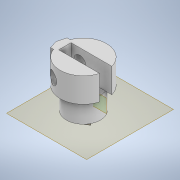
# Autodesk Inventor part: handle_base
Saved by Autodesk Inventor 2021 (Build 250183000, 183)
## iProperties
Created: 2021-03-06
Part Number: handle_base
Material: Generic
Document SubType Name: Modeling
Designer: ben
Density: 1 g/cm^3
Appearance: Default
Mass: 193.865 g
Surface Area: 332.78 cm^2
Volume: 193.865 cm^3
Author: ben
Autodesk Inventor part; units mm, degrees
ref_plane "YZ Plane" through (0, 0, 0) normal (1, 0, 0) x (0, 1, 0)
ref_plane "XZ Plane" through (0, 0, 0) normal (0, 1, 0) x (-1, 0, 0)
ref_plane "XY Plane" through (0, 0, 0) normal (0, 0, 1) x (1, 0, 0)
ref_plane "Work Plane1" through (-35, 22.5, -35) normal (0, 0, 1) x (1, 0, 0)
sketch "Sketch1" plane through (-35, 22.5, -35) normal (0, 0, 1) x (1, 0, 0)
  circle A0 centre (35, -42) radius 27.5
  circle A1 centre (35, -42) radius 6
  point P0 (35, -22.5)
  dimension "d0" = 55
  dimension "d24" = 12
  constraints: 2 centre point, 1 coincident
  measures "d0" diameter of A0
  measures "d24" diameter of A1
ref_plane "Work Plane2" through (0, -19.5, 0) normal (0, 0, 1) x (1, 0, 0)
sketch "Sketch2" plane through (0, -19.5, 0) normal (0, 0, 1) x (1, 0, 0)
  arc A0 (-36.1421, -10) -> (-36.1421, 10) centre (0, 0) ccw
  line L0 (30, -10) -> (-36.1421, -10)
  line L1 (-36.1421, 10) -> (30, 10)
  line L2 (30, 10) -> (30, -10)
  line L3 (34.9857, -13.5) -> (39.9857, -13.5)
  line L4 (39.9857, -13.5) -> (39.9857, 13.5)
  line L5 (39.9857, 13.5) -> (34.9857, 13.5)
  line L6 (34.9857, 13.5) -> (34.9857, -13.5)
  line L7 (39.9857, -13.5) -> (43.6938, 0)
  line L8 (43.6938, 0) -> (39.9857, 13.5)
  point P0 (0, 19.5)
  dimension "d3" = 75
  dimension "d40" = 5
  dimension "d41" = 27
  dimension "d44" = 14
  constraints: 18 end point, 4 horizontal, 4 point on circle, 3 parallel, 1 centre point, 1 perpendicular, 1 vertical, 1 other
  measures "d3" diameter of A0
  measures "d40" distance of L3.start L3.end
  measures "d41" distance of L5.end L3.start
  measures "d44" distance of L3.end L7.end
extrude "Extrusion2" add sketch "Sketch2" along normal blind 40
ref_plane "Work Plane3" through (-36.1421, -9.5, 0) normal (0, -1, 0) x (1, 0, 0)
sketch "Sketch4" plane through (-36.1421, -9.5, 0) normal (0, -1, 0) x (1, 0, 0)
  line L0 (0, 0) -> (10.5247, 0) projected
  point P0 (36.1421, 0)
  point P1 (51.9367, 20)
hole "Hole2" at (15.7946, -9.5, 20) direction (0, 1, 0) diameter 19.05 end through all both
extrude "Extrusion3" add sketch "Sketch1" along normal blind 35
sketch "Sketch8" plane through (0, -19.5, -35) normal (0, 0, -1) x (-1, 0, 0)
  circle A0 centre (0, 0) radius 6 projected
  circle A1 centre (0, 0) radius 6 projected
  line L0 (-6, 10.3923) -> (12, 0)
  line L1 (12, 0) -> (-6, -10.3923)
  line L2 (-6, -10.3923) -> (-6, 10.3923)
  point P0 (0, 19.5)
  point P1 (-6, 0)
  constraints: 6 end point, 1 coincident, 1 horizontal alignment, 1 midpoint, 8 other
extrude "Extrusion5" add sketch "Sketch8" along normal blind 15
sketch "Sketch9" plane through (0, -19.5, -35) normal (0, 0, -1) x (-1, 0, 0)
  circle A0 centre (0, 0) radius 6 projected
  line L0 (-3.7474, -4.6858) -> (-3.7474, 4.6858)
  point P0 (0, 19.5)
  constraints: 2 end point, 2 point on circle, 2 vertical
extrude "Extrusion6" add sketch "Sketch9" against normal blind 10 contours A0 L0 picked at (-0.4983, 0)
body "Solid1"
